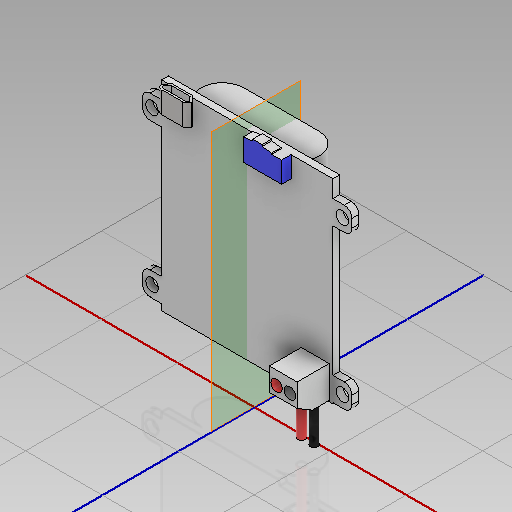
# Autodesk Inventor part: ЛЦМК000002.00.00.00.00.12
Saved by Autodesk Inventor 2021.2 (Build 252289000, 289)
## iProperties
Created: 2025-11-03
Part Number: ЛЦМК000002.00.00.00.00.12
Material: Типовые
Document SubType Name: Modeling
Designer: Захаров
Density: 1 g/cm^3
Appearance: По умолчанию
Author: Захаров
Autodesk Inventor part; units mm, degrees
ref_plane "YZ Plane" through (0, 0, 0) normal (1, 0, 0) x (0, 1, 0)
ref_plane "XZ Plane" through (0, 0, 0) normal (0, 1, 0) x (-1, 0, 0)
ref_plane "XY Plane" through (0, 0, 0) normal (0, 0, 1) x (1, 0, 0)
sketch "Эскиз1" plane through (0, 0, 0) normal (0, 0, 1) x (1, 0, 0)
  line L0 (22.5, -26.25) -> (-22.5, -26.25)
  line L1 (-22.5, -26.25) -> (-22.5, 26.25)
  line L2 (-22.5, 26.25) -> (22.5, 26.25)
  line L3 (22.5, 26.25) -> (22.5, -26.25)
  line L4 (22.5, -26.25) -> (-22.5, 26.25) construction
  line L5 (-22.5, -26.25) -> (22.5, 26.25) construction
  point P0 (0, 0)
  dimension "d0" = 45
  dimension "d1" = 52.5
  constraints: 12 end point, 2 midpoint, 2 parallel, 1 horizontal, 1 perpendicular
  measures "d0" distance of L1.end L2.end
  measures "d1" distance of L0.end L1.end
extrude "Выдавливание1" add sketch "Эскиз1" along normal blind 1.8
sketch "Эскиз2" plane through (0, 0, 1.8) normal (0, 0, 1) x (1, 0, 0)
  line L0 (22.5, -26.25) -> (22.5, 26.25) projected
  line L1 (22.5, 21.75) -> (27.5, 21.75)
  line L2 (27.5, 21.75) -> (27.5, 15.55)
  line L3 (27.5, 15.55) -> (22.5, 15.55)
  line L4 (22.5, 15.55) -> (22.5, 21.75)
  line L5 (22.5, 26.25) -> (-22.5, 26.25) projected
  line L6 (22.5, -18.45) -> (27.5, -18.45)
  line L7 (27.5, -18.45) -> (27.5, -24.65)
  line L8 (27.5, -24.65) -> (22.5, -24.65)
  line L9 (22.5, -24.65) -> (22.5, -18.45)
  point P0 (0, 0)
  dimension "d4" = 4.5
  dimension "d5" = 6.2
  dimension "d6" = 5
  dimension "d9" = 40.2
  constraints: 16 end point, 2 parallel, 1 horizontal, 1 perpendicular, 1 point on line, 1 vertical, 8 other
  measures "d4" distance between parallel lines of L5 L1
  measures "d5" distance of L1.end L2.end
  measures "d6" distance of L1.start L1.end
  measures "d9" distance of L1.start L6.start
extrude "Выдавливание2" add sketch "Эскиз2" against normal blind 1.8
sketch "Эскиз3" plane through (0, 0, 1.8) normal (0, 0, 1) x (1, 0, 0)
  line L0 (22.5, 26.25) -> (-22.5, 26.25) projected
  line L1 (-22.5, 26.25) -> (-22.5, -26.25) projected
  line L2 (-22.5, -26.25) -> (22.5, -26.25) projected
  line L3 (22.5, -26.25) -> (22.5, -24.65) projected
  line L4 (22.5, -24.65) -> (27.5, -24.65) projected
  line L5 (27.5, -24.65) -> (27.5, -18.45) projected
  line L6 (27.5, -18.45) -> (22.5, -18.45) projected
  line L7 (22.5, -18.45) -> (22.5, 15.55) projected
  line L8 (22.5, 15.55) -> (27.5, 15.55) projected
  line L9 (27.5, 15.55) -> (27.5, 21.75) projected
  line L10 (27.5, 21.75) -> (22.5, 21.75) projected
  line L11 (22.5, 21.75) -> (22.5, 26.25) projected
  circle A0 centre (25, 18.65) radius 1.65
  circle A1 centre (25, -21.55) radius 1.65
  point P0 (0, 0)
  dimension "d16" = 3.3
  dimension "d19" = 40.2
  constraints: 2 centre point, 1 vertical, 2 other
  measures "d16" diameter of A0
  measures "d19" distance of A0.centre A1.centre
extrude "Выдавливание3" cut sketch "Эскиз3" against normal blind 1.8 contours A0 | A1
fillet "Сопряжение1" radius 2 4 edges at (27.5, 15.55, 0.9) (27.5, 21.75, 0.9) (27.5, -18.45, 0.9) (27.5, -24.65, 0.9)
mirror "Зеркальное отражение1" about plane through (0, 0, 0) normal (1, 0, 0) of "Выдавливание3", "Сопряжение1", "Выдавливание2"
sketch "Эскиз4" plane through (0, 0, 1.8) normal (0, 0, 1) x (1, 0, 0)
  line L0 (14.2, -24.65) -> (21.5, -24.65)
  line L1 (21.5, -16.25) -> (14.2, -16.25)
  line L2 (14.2, -16.25) -> (14.2, -24.65)
  line L3 (-22.5, -26.25) -> (22.5, -26.25) projected
  line L4 (27.5, -22.65) -> (27.5, -20.45) projected
  line L5 (21.5, -16.25) -> (21.5, -24.65)
  line L6 (22.5, -18.45) -> (22.5, 15.55) projected
  point P0 (0, 0)
  point P1 (22.5, -24.65)
  dimension "d27" = 10
  dimension "d48" = 7.3
  dimension "d49" = 8.3
  constraints: 8 end point, 1 horizontal, 1 parallel, 1 perpendicular
  measures "d27" distance between parallel lines of L3 L1
  measures "d48" distance of L1.start L1.end
  measures "d49" distance between parallel lines of L6 L2
extrude "Выдавливание4" add sketch "Эскиз4" along normal blind 8.4
sketch "Эскиз5" plane through (21.5, -18.45, 0) normal (1, 0, 0) x (0, 0, -1)
  line L0 (-1.8, 0) -> (0, 0) projected
  line L1 (0, 0) -> (0, 34) projected
  line L2 (0, 34) -> (-1.8, 34) projected
  line L3 (-1.8, -7.8) -> (-1.8, -6.2) projected
  line L4 (-1.8, 0) -> (-1.8, 34) projected
  line L5 (-6.2, -6.2) -> (-10.2, -3.8)
  line L6 (0, -6.2) -> (-1.8, -6.2) projected
  line L7 (0, -7.8) -> (-1.8, -7.8) projected
  line L8 (0, -7.8) -> (0, -6.2) projected
  line L9 (-1.8, 40.2) -> (0, 40.2) projected
  line L10 (0, 40.2) -> (0, 44.7) projected
  line L11 (0, 44.7) -> (-1.8, 44.7) projected
  line L12 (-1.8, 40.2) -> (-1.8, 44.7) projected
  line L13 (-10.2, -3.8) -> (-10.2, -6.2)
  line L14 (-10.2, -6.2) -> (-6.2, -6.2)
  line L15 (-1.8, 2.2) -> (-10.2, 2.2) projected
  dimension "d50" = 6
  constraints: 6 end point
  measures "d50" distance from line of L15 L5.end
extrude "Выдавливание5" cut sketch "Эскиз5" against normal through all contours L14 L13 L5
sketch "Эскиз6" plane through (0, 0, 10.2) normal (0, 0, 1) x (1, 0, 0)
  circle A0 centre (16.1, -19.75) radius 1.5
  line L0 (14.2, -16.25) -> (14.2, -24.65) projected
  line L1 (21.5, -16.25) -> (14.2, -16.25) projected
  circle A1 centre (19.6, -19.75) radius 1.5
  line L2 (21.5, -22.25) -> (21.5, -16.25) projected
  point P0 (0, 0)
  point P1 (14.2, -22.25)
  dimension "d35" = 3
  dimension "d36" = 1.9
  dimension "d37" = 3.5
  dimension "d51" = 1.9
  constraints: 2 centre point, 1 equal radius, 1 horizontal alignment
  measures "d35" diameter of A0
  measures "d36" distance from line of L0 A0.centre
  measures "d37" distance from line of L1 A0.centre
  measures "d51" distance from line of L2 A1.centre
extrude "Выдавливание6" cut sketch "Эскиз6" against normal blind 4
sketch "Эскиз7" plane through (14.2, -24.65, 1.8) normal (0, -1, 0) x (1, 0, 0)
  line L0 (0.5, 3.9) -> (3.5, 3.9)
  line L1 (3.5, 3.9) -> (3.5, -0.1)
  line L2 (3.5, -0.1) -> (0.5, -0.1)
  line L3 (0.5, -0.1) -> (0.5, 3.9)
  line L4 (0, 0) -> (0, 8.4) projected
  line L5 (7.3, 4.4) -> (0, 4.4) projected
  line L6 (0, 8.4) -> (7.3, 8.4) projected
  line L7 (4, 3.9) -> (7, 3.9)
  line L8 (7, 3.9) -> (7, -0.1)
  line L9 (7, -0.1) -> (4, -0.1)
  line L10 (4, -0.1) -> (4, 3.9)
  point P0 (-14.2, -1.8)
  point P1 (5.5, -0.1)
  point P2 (2, -0.1)
  dimension "d42" = 3
  dimension "d43" = 4
  dimension "d44" = 0.5
  dimension "d46" = 4.5
  dimension "d47" = 0.5
  constraints: 16 end point, 4 parallel, 2 equal length, 2 horizontal, 2 midpoint, 2 perpendicular, 1 horizontal alignment
  measures "d42" distance of L1.end L2.end
  measures "d43" distance of L0.end L1.end
  measures "d44" distance between parallel lines of L4 L3
  measures "d46" distance between parallel lines of L6 L0
  measures "d47" distance between parallel lines of L1 L10
extrude "Выдавливание7" cut sketch "Эскиз7" against normal blind 4
sketch "Эскиз8" plane through (0, 0, 1.8) normal (0, 0, 1) x (1, 0, 0)
  line L0 (22.5, -24.9377) -> (8.5, -24.9377)
  line L1 (-22.5, -26.25) -> (22.5, -26.25) projected
  line L2 (22.5, -26.25) -> (22.5, -24.65) projected
  line L3 (8.5, -24.9377) -> (8.2, -26.25)
  point P0 (0, 0)
  dimension "d55" = 14
  dimension "d56" = 0.3
  constraints: 4 end point, 2 point on line, 1 horizontal
  measures "d55" distance of L0.start L0.end
  measures "d56" horizontal distance of L0.end L3.end
extrude "Выдавливание8" cut sketch "Эскиз8" against normal blind 4
sketch "Эскиз9" plane through (14.2, -24.65, 6.2) normal (0, -1, 0) x (1, 0, 0)
  circle A0 centre (2.0513, -2.4) radius 1
  circle A1 centre (5.3513, -2.4) radius 1
  line L0 (-5.7, -4.4) -> (8.3, -4.4) projected
  point P0 (-14.2, -6.2)
  dimension "d59" = 2
  dimension "d60" = 2
  dimension "d61" = 3.3
  dimension "d62" = 2
  constraints: 2 centre point, 1 horizontal alignment
  measures "d59" diameter of A0
  measures "d60" diameter of A1
  measures "d61" distance of A0.centre A1.centre
  measures "d62" distance from line of L0 A0.centre
extrude "Выдавливание9" add sketch "Эскиз9" along normal blind 10 and the other way blind 4.25
sketch "Эскиз10" plane through (0, 0, 1.8) normal (0, 0, 1) x (1, 0, 0)
  line L0 (-21, 26.75) -> (-13, 26.75)
  line L1 (-13, 26.75) -> (-13, 21.05)
  line L2 (-13, 21.05) -> (-21, 21.05)
  line L3 (-21, 21.05) -> (-21, 26.75)
  line L4 (22.5, 26.25) -> (-22.5, 26.25) projected
  line L5 (-22.5, 26.25) -> (-22.5, 21.75) projected
  point P0 (0, 0)
  dimension "d67" = 8
  dimension "d68" = 5.7
  dimension "d69" = 0.5
  dimension "d70" = 9.5
  constraints: 8 end point, 2 parallel, 1 horizontal, 1 perpendicular
  measures "d67" distance of L1.end L2.end
  measures "d68" distance of L0.end L1.end
  measures "d69" distance between parallel lines of L4 L0
  measures "d70" distance between parallel lines of L5 L1
extrude "Выдавливание10" add sketch "Эскиз10" along normal blind 2.7
sketch "Эскиз11" plane through (-21, 26.75, 1.8) normal (0, 1, 0) x (1, 0, 0)
  line L0 (8, -2.7) -> (0, -2.7) projected
  line L1 (8, 0) -> (8, -2.7) projected
  arc A0 (6.8162, -2.7) -> (8, -1.5162) centre (6.8162, -1.5162) ccw
  line L2 (8, -1.5162) -> (6.7126, 0)
  line L3 (8, 0) -> (0, 0) projected
  line L4 (8, 0) -> (0, 0) projected
  line L5 (0, 0) -> (0, -2.7) projected
  line L6 (8, -2.7) -> (0, -2.7) projected
  line L7 (8, 0) -> (8, -2.7) projected
  line L8 (4, -2.7) -> (4, -0.3754) construction
  arc A1 (0, -1.5162) -> (1.1838, -2.7) centre (1.1838, -1.5162) ccw
  line L9 (0, -1.5162) -> (1.2874, 0)
  point P0 (21, 1.8)
  point P1 (0, -1.5162)
  point P2 (0, -1.5162)
  point P3 (1.2874, 0)
  point P4 (1.1838, -2.7)
  constraints: 6 end point, 4 point on circle, 4 symmetric about line, 3 point on line, 2 centre point, 2 tangent, 1 midpoint, 1 vertical, 1 other
extrude "Выдавливание11" cut sketch "Эскиз11" against normal through all contours L0 A0 L1 | L2 L3 L1 | L0 L5 A1 | L5 L3 L9
sketch "Эскиз12" plane through (-19.7126, 26.75, 1.8) normal (0, 1, 0) x (1, 0, 0)
  line L0 (6.7126, -1.5162) -> (5.4252, 0) projected
  line L1 (5.4252, 0) -> (0, 0) projected
  line L2 (0, 0) -> (-1.2874, -1.5162) projected
  arc A0 (-1.2874, -1.5162) -> (-0.1037, -2.7) centre (-0.1037, -1.5162) ccw projected
  line L3 (5.5288, -2.7) -> (-0.1037, -2.7) projected
  arc A1 (5.5288, -2.7) -> (6.7126, -1.5162) centre (5.5288, -1.5162) ccw projected
  arc A2 (-0.7682, -1.6772) -> (-0.1037, -2.2) centre (-0.1037, -1.5162) ccw
  line L4 (-0.7682, -1.6772) -> (0.2314, -0.5)
  line L5 (0.2314, -0.5) -> (5.1938, -0.5)
  line L6 (5.1938, -0.5) -> (6.1934, -1.6772)
  arc A3 (5.5288, -2.2) -> (6.1934, -1.6772) centre (5.5288, -1.5162) ccw
  line L7 (5.5288, -2.2) -> (-0.1037, -2.2)
  point P0 (19.7126, 1.8)
  dimension "d4" = 4.5
  dimension "d5" = 6.2
  dimension "d6" = 5
  dimension "d9" = 40.2
  dimension "d75" = 0.5
  constraints: 8 end point, 4 point on circle, 2 centre point, 5 other
  measures "d75" distance between parallel lines of L3 L7
extrude "Выдавливание12" cut sketch "Эскиз12" against normal blind 4.5 contours L4 L5 L6 A3 L7 A2
sketch "Эскиз13" plane through (0, 0, 1.8) normal (0, 0, 1) x (1, 0, 0)
  line L0 (1.5, 27.25) -> (11.5, 27.25)
  line L1 (11.5, 27.25) -> (11.5, 20.75)
  line L2 (11.5, 20.75) -> (1.5, 20.75)
  line L3 (1.5, 20.75) -> (1.5, 27.25)
  line L4 (22.5, 26.25) -> (-14.2874, 26.25) projected
  line L5 (22.5, 21.75) -> (22.5, 26.25) projected
  point P0 (0, 0)
  dimension "d78" = 10
  dimension "d79" = 6.5
  dimension "d80" = 1
  dimension "d81" = 21
  constraints: 8 end point, 2 parallel, 1 horizontal, 1 perpendicular
  measures "d78" distance of L1.end L2.end
  measures "d79" distance of L0.end L1.end
  measures "d80" distance between parallel lines of L4 L0
  measures "d81" distance between parallel lines of L5 L3
extrude "Выдавливание13" add sketch "Эскиз13" along normal blind 2.5
sketch "Эскиз14" plane through (0, 0, 4.3) normal (0, 0, 1) x (1, 0, 0)
  line L0 (22.5, 26.25) -> (-22.5, 26.25) projected
  line L1 (1.5, 27.25) -> (1.5, 20.75) projected
  line L2 (1.5, 26.25) -> (1.5, 26.55)
  line L3 (1.5, 26.55) -> (3.9858, 26.8164)
  line L4 (3.9858, 26.8164) -> (3.9393, 27.25)
  line L5 (11.5, 27.25) -> (1.5, 27.25) projected
  line L6 (3.9393, 27.25) -> (6.4393, 27.25)
  line L7 (11.5, 27.25) -> (1.5, 27.25) projected
  line L8 (5.1893, 27.25) -> (5.1893, 26.4) construction
  line L9 (8.8786, 26.25) -> (8.8786, 26.55)
  line L10 (8.8786, 26.55) -> (6.3928, 26.8164)
  line L11 (6.3928, 26.8164) -> (6.4393, 27.25)
  line L12 (11.5, 20.75) -> (11.5, 27.25) projected
  point P0 (0, 0)
  point P1 (11.5, 26.25)
  dimension "d84" = 0.3
  dimension "d85" = 2.5
  dimension "d86" = 2.5
  dimension "d87" = 1.25
  constraints: 16 end point, 6 point on line, 4 symmetric about line, 1 perpendicular, 1 vertical
  measures "d84" distance of L2.start L2.end
  measures "d85" distance of L2.end L3.end
  measures "d86" distance of L4.end L6.end
  measures "d87" distance of L4.end L8.start
extrude "Выдавливание14" cut sketch "Эскиз14" against normal blind 2.5 contours L9 L10 L11 L5 L12 L0 | L1 L5 L4 L3
sketch "Эскиз15" plane through (-22.5, -26.25, 0) normal (0, -1, 0) x (1, 0, 0)
  line L0 (34, -5.6) -> (3, -5.6) construction
  line L1 (28.4, 0) -> (8.6, 0)
  line L2 (8.6, -11.2) -> (28.4, -11.2)
  arc A0 (28.4, -11.2) -> (28.4, 0) centre (28.4, -5.6) ccw
  arc A1 (8.6, 0) -> (8.6, -11.2) centre (8.6, -5.6) ccw
  line L3 (0, 1.8) -> (30.7, 1.8) projected
  line L4 (0, 0) -> (30.7, 0) projected
  point P0 (22.5, 0)
  point P1 (18.5, -5.6)
  point P2 (15.35, 0)
  point P3 (45, 0)
  dimension "d90" = 31
  dimension "d91" = 13
  dimension "d95" = 3
  constraints: 8 end point, 6 point on circle, 4 tangent, 3 point on line, 2 centre point, 2 midpoint, 1 horizontal, 1 parallel
  measures "d90" distance of L0.start L0.end
  measures "d91" distance between parallel lines of L3 L2
  measures "d95" horizontal distance of L4.start L0.end
extrude "Выдавливание15" add sketch "Эскиз15" against normal blind 48.5
ref_plane "РабПлоскость1" through (0, 0, 0) normal (1, 0, 0) x (0, 1, 0)
